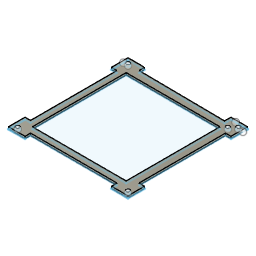
Polarizer Frame v3 (Autodesk Fusion 360 design; units mm, degrees)
Autodesk Fusion 360 part; units mm, degrees
sketch "polarizer frame" plane through (0, 0, 0) normal (0, 0, 1) x (1, 0, 0)
  line L0 (130, 48) -> (130, -54)
  line L1 (130, -54) -> (232, -54)
  line L2 (234, 63) -> (247, 63)
  line L3 (247, -54) -> (247, -67)
  line L4 (117, 63) -> (117, 58)
  circle A0 centre (122, 58) radius 2
  line L5 (247, 63) -> (247, 58)
  circle A1 centre (242, 58) radius 2
  line L6 (247, -67) -> (242, -67)
  circle A2 centre (242, -62) radius 2
  line L7 (117, -67) -> (122, -67)
  circle A3 centre (122, -62) radius 2
  circle A4 centre (236.3431, 52.3431) radius 2
  line L8 (232, 48) -> (232, -54)
  line L9 (232, 48) -> (130, 48)
  line L10 (135, 63) -> (135, 59)
  line L11 (247, 63) -> (229, 63)
  line L12 (229, 63) -> (229, 59)
  line L13 (135, 59) -> (135, 57)
  line L14 (135, 57) -> (229, 56)
  line L15 (229, 56) -> (229, 59)
  line L16 (117, 63) -> (135, 63)
  line L17 (229, 63) -> (247, 63)
  line L18 (117, 63) -> (117, 45)
  line L19 (117, 45) -> (123, 45)
  line L20 (117, -67) -> (117, -49)
  line L21 (117, -49) -> (123, -49)
  line L22 (123, -49) -> (123, 45)
  line L23 (117, -67) -> (117, -49)
  line L24 (117, 45) -> (117, 63)
  line L25 (247, 63) -> (247, 45)
  line L26 (247, -67) -> (247, -49)
  line L27 (247, -49) -> (241, -49)
  line L28 (247, 45) -> (241, 45)
  line L29 (241, 45) -> (241, -49)
  line L30 (247, 63) -> (247, 45)
  line L31 (247, -49) -> (247, -54)
  line L32 (117, -67) -> (135, -67)
  line L33 (247, -67) -> (229, -67)
  line L34 (135, -67) -> (135, -61)
  line L35 (135, -61) -> (229, -61)
  line L36 (229, -61) -> (229, -67)
  line L37 (247, -67) -> (229, -67)
  line L38 (135, -67) -> (117, -67)
  dimension "d21" = 13
  dimension "d22" = 13
  dimension "d23" = 130
  dimension "d24" = 130
  dimension "d25" = 5
  dimension "d26" = 4
  dimension "d27" = 5
  dimension "d28" = 5
  dimension "d29" = 4
  dimension "d30" = 4
  dimension "d31" = 4
  dimension "d43" = 8
  dimension "d44" = 4
  dimension "d47" = 18
  dimension "d48" = 4
  dimension "d49" = 18
  dimension "d50" = 18
  dimension "d51" = 6
  dimension "d52" = 18
  dimension "d53" = 18
  dimension "d54" = 6
  dimension "d55" = 6
  dimension "d56" = 18
  dimension "d57" = 18
  dimension "d58" = 6
  constraint perpendicular L0 L1
  constraint perpendicular L3 L37
  constraint perpendicular L4 L16
  constraint perpendicular L5 L16
  constraint coincident L6.end L37
  constraint coincident L7.end L37
  constraint perpendicular L7 L23
  constraint perpendicular L1 L8
  constraint perpendicular L0 L9
  constraint perpendicular L10 L16
  constraint coincident L11.end L16
  constraint perpendicular L11 L30
  constraint perpendicular L11 L12
  constraint collinear L16 L17
  constraint coincident L18.end L23
  constraint perpendicular L19 L23
  constraint perpendicular L20 L37
  constraint perpendicular L20 L21
  constraint collinear L23 L24
  constraint perpendicular L17 L25
  constraint perpendicular L6 L26
  constraint perpendicular L26 L27
  constraint perpendicular L25 L28
  constraint perpendicular L27 L29
  constraint collinear L30 L31
  constraint perpendicular L23 L32
  constraint perpendicular L26 L33
  constraint perpendicular L32 L34
  constraint perpendicular L34 L35
  constraint perpendicular L33 L36
  constraint collinear L37 L38
  measures "d21" distance of L2.start L2.end
  measures "d22" distance of L3.start L3.end
  measures "d23" distance of L3.end L7.start
  measures "d24" distance of L7.start L4.start
  measures "d25" distance of L4.start L4.end
  measures "d26" diameter of A0
  measures "d27" distance of L2.end L5.end
  measures "d28" distance of L5.end A1.centre
  measures "d29" diameter of A1
  measures "d30" diameter of A2
  measures "d31" diameter of A3
  measures "d43" distance of A1.centre A4.centre
  measures "d44" diameter of A4
  measures "d47" distance of L2.end L11.end
  measures "d48" distance of L11.end L12.end
  measures "d49" distance of L4.start L18.end
  measures "d50" distance of L7.start L20.end
  measures "d51" distance of L20.end L21.end
  measures "d52" distance of L2.end L25.end
  measures "d53" distance of L3.end L26.end
  measures "d54" distance of L26.end L27.end
  measures "d55" distance of L25.end L28.end
  measures "d56" distance of L7.start L32.end
  measures "d57" distance of L3.end L33.end
  measures "d58" distance of L32.end L34.end
extrude "Extrude7" add sketch "polarizer frame" along normal blind 2.25
named bodies: "polarizer frame"
